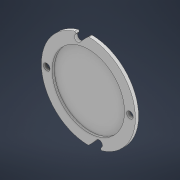
# Autodesk Inventor part: kanure_01
Saved by Autodesk Inventor 2022 (Build 260153000, 153)
## iProperties
Created: 2023-06-03
Part Number: kanure_01
Material: 一般
Document SubType Name: Modeling
Designer: nyxeon
Density: 1 g/cm^3
Appearance: 既定
Author: nyxeon
Autodesk Inventor part; units mm, degrees
ref_plane "YZ Plane" through (0, 0, 0) normal (1, 0, 0) x (0, 1, 0)
ref_plane "XZ Plane" through (0, 0, 0) normal (0, 1, 0) x (-1, 0, 0)
ref_plane "XY Plane" through (0, 0, 0) normal (0, 0, 1) x (1, 0, 0)
sketch "スケッチ1" plane through (0, 0, 0) normal (0, 0, 1) x (1, 0, 0)
  circle A0 centre (0, 0) radius 33.5 construction
  circle A1 centre (0, 0) radius 43.5
  dimension "d0" = 67
  dimension "d1" = 87
  constraints: 2 centre point, 2 coincident
  measures "d0" diameter of A0
  measures "d1" diameter of A1
extrude "押し出し1" add sketch "スケッチ1" along normal blind 1
sketch "スケッチ2" plane through (0, 0, 1) normal (0, 0, 1) x (1, 0, 0)
  circle A0 centre (0, 0) radius 33.5
  circle A1 centre (0, 0) radius 43.5 projected
  dimension "d4" = 67
  constraints: 1 centre point, 1 coincident
  measures "d4" diameter of A0
extrude "押し出し2" add sketch "スケッチ2" along normal blind 2
sketch "スケッチ4" plane through (0, 0, 3) normal (0, 0, 1) x (1, 0, 0)
  circle A0 centre (0, 0) radius 33.5 construction
  circle A1 centre (0, 0) radius 43.5 construction
  line L0 (0, 0) -> (33.5, 0) construction
  line L1 (33.5, 0) -> (43.5, 0) construction
  circle A2 centre (0, 0) radius 33.5 construction
  line L2 (0, 0) -> (-33.5, 0) construction
  circle A3 centre (0, 0) radius 43.5 construction
  line L3 (-43.5, 0) -> (-33.5, 0) construction
  circle A4 centre (38.5, 0) radius 3.05
  circle A5 centre (-38.5, 0) radius 3.05
  circle A6 centre (0, 0) radius 38.5 construction
  circle A7 centre (-9.9645, 37.1881) radius 3.05 construction
  arc A8 (-3.4944, 44.3648) -> (-9.9645, 37.1881) centre (38.5, 0) ccw construction
  line L4 (38.5, 0) -> (-9.9645, 37.1881) construction
  line L5 (-9.9645, 37.1881) -> (-12.3843, 39.0449) construction
  arc A9 (0.0788, 43.4999) -> (-7.5448, 35.3314) centre (38.5, 0) ccw
  arc A10 (-9.6001, 42.4274) -> (-12.3843, 39.0449) centre (38.5, 0) ccw
  arc A11 (-12.3843, 39.0449) -> (-7.5448, 35.3314) centre (-9.9645, 37.1881) ccw
  arc A12 (0.0788, 43.4999) -> (-9.6001, 42.4274) centre (0, 0) ccw
  circle A13 centre (9.9645, -37.1881) radius 3.05 construction
  line L6 (-38.5, 0) -> (9.9645, -37.1881) construction
  line L7 (9.9645, -37.1881) -> (12.3843, -39.0449) construction
  arc A14 (-0.0788, -43.4999) -> (7.5448, -35.3314) centre (-38.5, 0) ccw
  arc A15 (9.6001, -42.4274) -> (12.3843, -39.0449) centre (-38.5, 0) ccw
  arc A16 (12.3843, -39.0449) -> (7.5448, -35.3314) centre (9.9645, -37.1881) ccw
  arc A17 (-0.0788, -43.4999) -> (9.6001, -42.4274) centre (0, 0) ccw
  line L8 (-9.9645, 37.1881) -> (9.9645, -37.1881) construction
  dimension "d7" = 6.1
  dimension "d8" = 3.05
  dimension "d15" = 105
  constraints: 31 point on circle, 18 end point, 14 centre point, 11 coincident, 7 point on line, 3 midpoint, 2 equal radius, 1 collinear, 1 horizontal, 1 horizontal alignment, 1 other
  measures "d7" diameter of A4
  measures "d8" radius of A11
  measures "d15" angle of L0 L8
extrude "押し出し3" cut sketch "スケッチ4" against normal through all
fillet "フィレット1" radius 1 4 edges at (-9.6001, 42.4274, 1.5) (0.0788, 43.4999, 1.5) (-0.0788, -43.4999, 1.5) (9.6001, -42.4274, 1.5)
